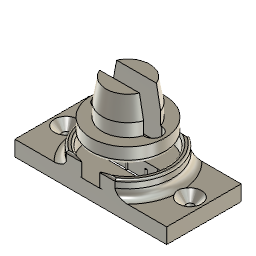
Lampy_Mag v1 (Autodesk Fusion 360 design; units mm, degrees)
Autodesk Fusion 360 part; units mm, degrees
note: some values were not read from the file. Chosen so that the rebuilt part matches the saved one: which face or edge a step refers to; which pieces of a blend or face edit are solid. Set by a fixed rule: which sketch regions a step uses.
sketch "Sketch1" plane through (0, 0, 0) normal (0, 0, 1) x (1, 0, 0)
  circle A0 centre (0, 0) radius 8
  circle A1 centre (0, 0) radius 6.6
  circle A2 centre (0, 0) radius 9.5
  line L0 (-5.5, 2.2) -> (5.5, 2.2)
  line L1 (5.5, 2.2) -> (5.5, -2.2)
  line L2 (5.5, -2.2) -> (-5.5, -2.2)
  line L3 (-5.5, -2.2) -> (-5.5, 2.2)
  line L4 (-5.5, 2.2) -> (5.5, -2.2) construction
  line L5 (5.5, 2.2) -> (-5.5, -2.2) construction
  line L6 (-2.7071, 2.2) -> (2.7071, -2.2) construction
  line L7 (2.7071, 2.2) -> (-2.7071, -2.2) construction
  line L8 (-6.5, 2.2) -> (6.5, 2.2)
  line L9 (6.5, 2.2) -> (6.5, -2.2)
  line L10 (6.5, -2.2) -> (-6.5, -2.2)
  line L11 (-6.5, -2.2) -> (-6.5, 2.2)
  line L12 (-6.5, 2.2) -> (6.5, -2.2) construction
  line L13 (6.5, 2.2) -> (-6.5, -2.2) construction
  circle A3 centre (5.5, 0) radius 2.2
  circle A4 centre (-5.5, 0) radius 2.2
  circle A5 centre (6.5, 0) radius 2.2
  circle A6 centre (-6.5, 0) radius 2.2
  line L14 (19.625, 9.625) -> (-19.625, 9.625)
  line L15 (-19.625, 9.625) -> (-19.625, -9.625)
  line L16 (-19.625, -9.625) -> (19.625, -9.625)
  line L17 (19.625, -9.625) -> (19.625, 9.625)
  line L18 (19.625, 9.625) -> (-19.625, -9.625) construction
  line L19 (-19.625, 9.625) -> (19.625, -9.625) construction
  circle A7 centre (-16, 0) radius 1
  circle A8 centre (16, 0) radius 1
  circle A9 centre (0, 0) radius 9.9
  circle A10 centre (0, 0) radius 11.5
  circle A11 centre (-2.5, 2.2) radius 0.25
  circle A12 centre (-2.5, -2.2) radius 0.25
  circle A13 centre (2.5, -2.2) radius 0.25
  circle A14 centre (2.5, 2.2) radius 0.25
  dimension "d1" = 16
  dimension "d2" = 13.2
  dimension "d8" = 19
  dimension "d17" = 11
  dimension "d18" = 4.4
  dimension "d19" = 4.4
  dimension "d20" = 13
  dimension "d21" = 4.4
  dimension "d22" = 4.4
  dimension "d23" = 4.4
  dimension "d24" = 4.4
  dimension "d31" = 4.4
  dimension "d32" = 39.25
  dimension "d33" = 19.25
  dimension "d34" = 2
  dimension "d35" = 2
  dimension "d36" = 19.8
  dimension "d37" = 23
  dimension "d54" = 0.5
  dimension "d55" = 0.5
  dimension "d56" = 0.5
  dimension "d57" = 0.5
  constraint coincident A0.centre A1.centre
  constraint concentric A0 A1
  constraint concentric A0 A2
  constraint horizontal L0
  constraint perpendicular L0 L1
  constraint parallel L0 L2
  constraint parallel L1 L3
  constraint coincident L4 A0.centre
  constraint coincident L5 A0.centre
  constraint coincident L6 A0.centre
  constraint coincident L7 A0.centre
  constraint horizontal L8
  constraint perpendicular L8 L9
  constraint parallel L8 L10
  constraint parallel L9 L11
  constraint coincident L12 A0.centre
  constraint coincident L13 A0.centre
  constraint midpoint L1 A3.centre
  constraint midpoint L3 A4.centre
  constraint midpoint L9 A5.centre
  constraint midpoint L11 A6.centre
  constraint horizontal L14
  constraint perpendicular L14 L15
  constraint parallel L14 L16
  constraint parallel L15 L17
  constraint coincident L18 A0.centre
  constraint coincident L19 A0.centre
  constraint concentric A1 A10
  constraint coincident L8 A11.centre
  constraint coincident L10 A12.centre
  constraint coincident L10 A13.centre
  constraint coincident L0 A14.centre
  measures "d1" diameter of A0
  measures "d2" diameter of A1
  measures "d8" diameter of A2
  measures "d17" distance of L1.end L2.end
  measures "d18" distance of L0.end L1.end
  measures "d19" distance of L7.start L6.end
  measures "d20" distance of L9.end L10.end
  measures "d21" diameter of A3
  measures "d22" diameter of A4
  measures "d23" diameter of A5
  measures "d24" diameter of A6
  measures "d31" distance of L8.start L10.end
  measures "d32" distance of L15.end L16.end
  measures "d33" distance of L14.end L15.end
  measures "d34" diameter of A7
  measures "d35" diameter of A8
  measures "d36" diameter of A9
  measures "d37" diameter of A10
  measures "d54" diameter of A11
  measures "d55" diameter of A12
  measures "d56" diameter of A13
  measures "d57" diameter of A14
extrude "Extrude3" add sketch "Sketch1" against normal blind 4 contours A0 L9 A3 A5 | A0 A5 | A0 A1 L8 A5 A6 | A0 A1 L10 A5 A6 | A0 L11 A4 A6 | A0 A6 | A1 L8 A5 | A1 L9 A3 A5 | A1 L9 A3 A5 | A1 L10 A5 | A1 L11 A4 A6 | A1 L8 A6 | A1 L9 A3 | A1 L9 A3 | A1 L10 A6 | A1 L11 A4 A6 | A1 L9 A3 | A1 L11 A4 | A1 L11 A4 | A1 L11 A4 | A2 makes body 1
extrude "Extrude4" add sketch "Sketch1" along normal blind 9 separate body contours A1 L0 L8 A11 A14 | A1 L8 A3 A5 | A1 A3 A5 | A1 L10 A3 A5 | A1 L2 L10 A12 A13 | A1 A3 A5 | A1 L8 A4 A6 | A1 A4 A6 | L0 L2 L8 L10 A3 A4 A11 A12 A13 A14 | L1 A3 A5 | L1 A3 A5 | A1 L1 L9 A3 A5 | A1 L9 | A1 L10 A4 A6 | A1 A4 A6 | L1 A3 A5 | L3 A4 A6 | L3 A4 A6 | A1 L11 | A1 L3 L11 A4 A6 | L0 L8 A14 | L0 L8 A14 | L1 A5 | L3 A4 A6 | L2 L10 A13 | L2 L10 A13 | L0 L8 A11 | L0 L8 A11 | L3 A6 | L2 L10 A12 | L2 L10 A12 makes body 2
chamfer "Chamfer1" distance 1 angle 80 1 edges at (-6.1534, -2.3867, 9) measured on face at (-3.4398, 0.6165, 9) on bodies 2
extrude "Extrude5" add sketch "Sketch1" against normal blind 4 contours A1 L0 L8 A11 A14 | A1 L8 A3 A5 | A1 A3 A5 | A1 L10 A3 A5 | A1 L2 L10 A12 A13 | A1 A3 A5 | A1 L8 A4 A6 | A1 A4 A6 | L0 L2 L8 L10 A3 A4 A11 A12 A13 A14 | L1 A3 A5 | L1 A3 A5 | A1 L1 L9 A3 A5 | A1 L9 | A1 L10 A4 A6 | A1 A4 A6 | L1 A3 A5 | L3 A4 A6 | L3 A4 A6 | A1 L11 | A1 L3 L11 A4 A6 | L0 L8 A14 | L0 L8 A14 | L1 A5 | L3 A4 A6 | L2 L10 A13 | L2 L10 A13 | L0 L8 A11 | L0 L8 A11 | L3 A6 | L2 L10 A12 | L2 L10 A12 bodies 1 2
extrude "Extrude6" cut sketch "Sketch1" along normal blind 9 and the other way blind 3 contours A0 L9 A3 A5 | A0 A5 | A0 L11 A4 A6 | A0 A6 | A1 L8 A5 | A1 L9 A3 A5 | A1 L9 A3 A5 | A1 L10 A5 | A1 L11 A4 A6 | A1 L8 A6 | A1 L8 A3 A5 | A1 L9 A3 | A1 L9 A3 | A1 A3 A5 | A1 L10 A6 | A1 L11 A4 A6 | A1 L9 A3 | A1 L10 A3 A5 | A1 A3 A5 | A1 L8 A4 A6 | A1 L11 A4 | A1 L11 A4 | A1 A4 A6 | L0 L2 L8 L10 A3 A4 A11 A12 A13 A14 | L1 A3 A5 | L1 A3 A5 | A1 L1 L9 A3 A5 | A1 L9 | A1 L10 A4 A6 | A1 L11 A4 | A1 A4 A6 | L1 A3 A5 | L3 A4 A6 | L3 A4 A6 | A1 L11 | A1 L3 L11 A4 A6 | L1 A5 | L3 A4 A6 | L0 L8 A11 | L3 A6 picked at (-2.5426, 2.1154) bodies 1
extrude "Extrude7" cut sketch "Sketch1" against normal blind 5 contours A1 L9 A3 | A1 L9 A3 | A1 L9 A3 | A1 L11 A4 | A1 L11 A4 | L0 L2 L8 L10 A3 A4 A11 A12 A13 A14 | L1 A3 A5 | L1 A3 A5 | A1 L1 L9 A3 A5 | A1 L9 | A1 L11 A4 | L1 A3 A5 | L3 A4 A6 | L3 A4 A6 | A1 L11 | A1 L3 L11 A4 A6 | L1 A5 | L3 A4 A6 | L0 L8 A11 | L3 A6 picked at (-2.5426, 2.1154) bodies 1
extrude "Extrude8" add sketch "Sketch1" against normal blind 4 separate body contours A0 L9 A3 A5 | A0 A5 | A0 A1 L8 A5 A6 | A0 A1 L10 A5 A6 | A0 L11 A4 A6 | A0 A6 | A1 L8 A5 | A1 L9 A3 A5 | A1 L9 A3 A5 | A1 L10 A5 | A1 L11 A4 A6 | A1 L8 A6 | A1 L0 L8 A11 A14 | A1 L8 A3 A5 | A1 L9 A3 | A1 L9 A3 | A1 A3 A5 | A1 L10 A6 | A1 L11 A4 A6 | A1 L9 A3 | A1 L10 A3 A5 | A1 L2 L10 A12 A13 | A1 A3 A5 | A1 L8 A4 A6 | A1 L11 A4 | A1 L11 A4 | A1 A4 A6 | L0 L2 L8 L10 A3 A4 A11 A12 A13 A14 | L1 A3 A5 | L1 A3 A5 | A1 L1 L9 A3 A5 | A1 L9 | A1 L10 A4 A6 | A1 L11 A4 | A1 A4 A6 | L1 A3 A5 | L3 A4 A6 | L3 A4 A6 | A1 L11 | A1 L3 L11 A4 A6 | L0 L8 A14 | L0 L8 A14 | L1 A5 | L3 A4 A6 | L2 L10 A13 | L2 L10 A13 | L0 L8 A11 | L0 L8 A11 | L3 A6 | L2 L10 A12 | L2 L10 A12 | A2 | L14 L16 L17 A10 | L14 L16 A9 A10 | L14 L16 A9 | L14 L15 L16 A10 | L14 L16 A9 A10 makes body 3
extrude "Extrude9" cut sketch "Sketch1" against normal blind 4 contours A0 L9 A3 A5 | A0 A5 | A0 L11 A4 A6 | A0 A6 | A1 L8 A5 | A1 L9 A3 A5 | A1 L9 A3 A5 | A1 L10 A5 | A1 L11 A4 A6 | A1 L8 A6 | A1 L8 A3 A5 | A1 L9 A3 | A1 L9 A3 | A1 A3 A5 | A1 L10 A6 | A1 L11 A4 A6 | A1 L9 A3 | A1 L10 A3 A5 | A1 A3 A5 | A1 L8 A4 A6 | A1 L11 A4 | A1 L11 A4 | A1 A4 A6 | L0 L2 L8 L10 A3 A4 A11 A12 A13 A14 | L1 A3 A5 | L1 A3 A5 | A1 L1 L9 A3 A5 | A1 L9 | A1 L10 A4 A6 | A1 L11 A4 | A1 A4 A6 | L1 A3 A5 | L3 A4 A6 | L3 A4 A6 | A1 L11 | A1 L3 L11 A4 A6 | L0 L8 A14 | L1 A5 | L3 A4 A6 | L2 L10 A13 | L0 L8 A11 | L3 A6 | L2 L10 A12 picked at (2.4583, 2.1278) picked at (2.5602, -2.1309) picked at (-2.5426, 2.1154) picked at (-2.4389, -2.1433) bodies 3
extrude "Extrude10" add sketch "Sketch1" against normal blind 1.5 contours A0 L9 A3 A5 | A0 A5 | A0 L11 A4 A6 | A0 A6 | A1 L8 A5 | A1 L9 A3 A5 | A1 L9 A3 A5 | A1 L10 A5 | A1 L11 A4 A6 | A1 L8 A6 | A1 L8 A3 A5 | A1 A3 A5 | A1 L10 A6 | A1 L11 A4 A6 | A1 L10 A3 A5 | A1 A3 A5 | A1 L8 A4 A6 | A1 A4 A6 | A1 L10 A4 A6 | A1 A4 A6 bodies 3
chamfer "Chamfer2" distance 2 angle 45 2 edges at (15.0677, 0.3616, 0) (-16.9323, 0.3616, 0) measured on face at (-1.8333, -7.15, 0) measured on face at (-1.8333, -7.15, 0) on bodies 3
extrude "Extrude11" add sketch "Sketch1" along normal blind 4 contours L14 L16 A9 A10 | L14 L16 A9 A10 bodies 3
fillet "Fillet1" radius 2 2 edges at (-11.5, 0, 0) (11.5, 0, 0) on bodies 3
fillet "Fillet2" radius 0.5 8 edges at (-9.9, 0, 4) (-11.5, 0, 4) (9.9, 0, 4) (11.5, 0, 4) (4.3054, -9.625, 4) (-4.3054, -9.625, 4) (-4.3054, 9.625, 4) (4.3054, 9.625, 4) on bodies 3
fillet "Fillet3" radius 1 1 edges at (-8.8571, 3.4353, -4) on bodies 1
delete_face "DeleteFace4" 1 faces at (2.2867, -2.0696, 0.3333) on bodies 1
delete_face "DeleteFace5" 1 faces at (-2.6654, -2.0126, 0.3333) on bodies 1
delete_face "DeleteFace6" 1 faces at (2.7133, 2.0696, 4.6667) on bodies 1
move_body "Move2" bodies 1 to x (1, 0, 0) y (0, 1, 0) z (0, 0, 1) at (0, 0, 10)
extrude "Extrude14" add sketch "Sketch1" against normal blind 4 contours L0 L8 A14 | L2 L10 A13 | L0 L8 A11 | L2 L10 A12 picked at (2.4583, 2.1278) picked at (2.5602, -2.1309) picked at (-2.5426, 2.1154) picked at (-2.4389, -2.1433) bodies 3
extrude "Extrude15" cut sketch "Sketch1" against normal blind 1.5 contours L0 L8 A14 | L2 L10 A13 | L0 L8 A11 | L2 L10 A12 picked at (2.4583, 2.1278) picked at (2.5602, -2.1309) picked at (-2.5426, 2.1154) picked at (-2.4389, -2.1433) bodies 3
